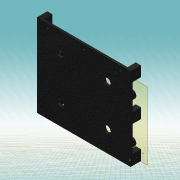
# Autodesk Inventor part: Down
Saved by Autodesk Inventor 2019 (Build 230136000, 136)
## iProperties
Created: 2024-12-30
Part Number: Down
Material: Nylon, molybdenum disulphide
Document SubType Name: Modeling
Designer: Familia CS
Density: 1.13 g/cm^3
Appearance: Black Cast
Author: Familia CS
Autodesk Inventor part; units mm, degrees
ref_plane "YZ Plane" through (0, 0, 0) normal (1, 0, 0) x (0, 1, 0)
ref_plane "XZ Plane" through (0, 0, 0) normal (0, 1, 0) x (-1, 0, 0)
ref_plane "XY Plane" through (0, 0, 0) normal (0, 0, 1) x (1, 0, 0)
ref_plane "Work Plane1" through (0, 0, 0) normal (0, 0, 1) x (1, 0, 0)
sketch "Sketch1" plane through (0, 0, 0) normal (0, 0, 1) x (1, 0, 0)
  circle A0 centre (-10, 5) radius 2 projected
  circle A1 centre (-80, 5) radius 2.426 projected
  circle A2 centre (-10, 45) radius 2 projected
  circle A3 centre (-80, 45) radius 2 projected
  circle A4 centre (-10, 5) radius 4
  circle A5 centre (-80, 5) radius 4
  circle A6 centre (-10, 45) radius 4
  circle A7 centre (-80, 45) radius 4
  point P0 (0, 0)
  dimension "d0" = 8
  dimension "d1" = 8
  dimension "d2" = 8
  dimension "d3" = 8
  constraints: 4 centre point, 4 coincident
  measures "d0" diameter of A4
  measures "d1" diameter of A5
  measures "d2" diameter of A6
  measures "d3" diameter of A7
extrude "Extrusion1" add sketch "Sketch1" along normal blind 10 contours A0 | A1 | A2 | A3 | A4 | A5 | A6 | A7
sketch "Sketch2" plane through (-10, 5, 10) normal (0, 0, 1) x (1, 0, 0)
  circle A0 centre (0, 0) radius 4 projected
  circle A1 centre (0, 0) radius 0.75
  circle A2 centre (-70, 0) radius 4 projected
  circle A3 centre (-70, 0) radius 0.75
  circle A4 centre (0, 40) radius 4 projected
  circle A5 centre (0, 40) radius 0.75
  circle A6 centre (-70, 40) radius 4 projected
  circle A7 centre (-70, 40) radius 0.75
  point P0 (10, -5)
  dimension "d6" = 1.5
  dimension "d7" = 1.5
  dimension "d8" = 1.5
  dimension "d9" = 1.5
  constraints: 4 centre point, 4 coincident
  measures "d6" diameter of A1
  measures "d7" diameter of A3
  measures "d8" diameter of A5
  measures "d9" diameter of A7
extrude "Extrusion2" cut sketch "Sketch2" against normal blind 10 contours A1 | A3 | A5 | A7
sketch "Sketch3" plane through (-10, 5, 10) normal (0, 0, 1) x (1, 0, 0)
  line L0 (-75, -10) -> (5, -10) projected
  line L1 (-80, 45) -> (-80, -5) projected
  line L2 (5, 50) -> (-75, 50) projected
  line L3 (10, -5) -> (10, 45) projected
  line L4 (-80.5, -10.5) -> (10.5, -10.5)
  line L5 (10.5, -10.5) -> (10.5, 70)
  line L6 (10.5, 70) -> (-80.5, 70)
  line L7 (-80.5, 70) -> (-80.5, -10.5)
  constraints: 8 end point, 2 parallel, 1 horizontal, 1 perpendicular
extrude "Extrusion3" add sketch "Sketch3" along normal blind 2
sketch "Sketch4" plane through (-10, 5, 12) normal (0, 0, 1) x (1, 0, 0)
  line L0 (-80.5, 70) -> (10.5, 70)
  circle A0 centre (-12.25, 9.625) radius 3.25
  circle A1 centre (-57.75, 9.625) radius 3.25
  circle A2 centre (-12.25, 49.875) radius 3.25
  circle A3 centre (-57.75, 50.6331) radius 3.25
  point P0 (10, -5)
  point P1 (10.5, -10.5)
  dimension "d18" = 6.5
  dimension "d19" = 6.5
  dimension "d20" = 6.5
  dimension "d21" = 6.5
  constraints: 4 centre point, 2 end point
  measures "d18" diameter of A0
  measures "d19" diameter of A1
  measures "d20" diameter of A2
  measures "d21" diameter of A3
extrude "Extrusion4" cut sketch "Sketch4" against normal blind 2
sketch "Sketch5" plane through (0.5, -5.5, 10) normal (1, 0, 0) x (0, 0, -1)
  point P0 (10, 5.5)
sketch "Sketch6" plane through (0.5, -5.5, 10) normal (1, 0, 0) x (0, 0, -1)
  point P0 (10, 5.5)
sketch "Sketch7" plane through (0.5, -5.5, 10) normal (1, 0, 0) x (0, 0, -1)
  line L0 (0, 0) -> (0, 80.5) projected
  line L1 (0, 0) -> (8, 0)
  line L2 (8, 0) -> (8, 10)
  line L3 (8, 10) -> (0, 10)
  line L4 (0, 10) -> (0, 0)
  circle A0 centre (4, 5) radius 0.75
  point P0 (10, 5.5)
  dimension "d24" = 8
  dimension "d25" = 10
  dimension "d26" = 1.5
  constraints: 8 end point, 2 parallel, 1 centre point, 1 horizontal, 1 perpendicular
  measures "d24" distance of L3.end L2.end
  measures "d25" distance of L2.end L1.end
  measures "d26" diameter of A0
extrude "Extrusion5" add sketch "Sketch7" against normal blind 5
sketch "Sketch8" plane through (-90.5, -5.5, 12) normal (0, -1, 0) x (1, 0, 0)
  line L0 (86, -10) -> (86, -2) projected
  line L1 (86, -10) -> (76, -10)
  line L2 (76, -10) -> (76, -2)
  line L3 (76, -2) -> (86, -2)
  line L4 (86, -2) -> (86, -10)
  circle A0 centre (81, -6) radius 0.75
  point P0 (90.5, -12)
  dimension "d29" = 10
  dimension "d30" = 8
  dimension "d31" = 1.5
  constraints: 8 end point, 2 parallel, 1 centre point, 1 horizontal, 1 perpendicular
  measures "d29" distance of L2.end L3.end
  measures "d30" distance of L1.end L2.end
  measures "d31" diameter of A0
extrude "Extrusion6" add sketch "Sketch8" against normal blind 5
fillet "Fillet1" radius 1 1 edges at (-14, 5, 10)
sketch "Sketch9" plane through (-90.5, -5.5, 12) normal (0, -1, 0) x (1, 0, 0)
  line L0 (0, -2) -> (76, -2) projected
  line L1 (0, -2) -> (10, -2)
  line L2 (10, -2) -> (10, -10)
  line L3 (10, -10) -> (0, -10)
  line L4 (0, -10) -> (0, -2)
  circle A0 centre (5, -6) radius 0.75
  point P0 (90.5, -12)
  dimension "d35" = 10
  dimension "d36" = 8
  dimension "d37" = 1.5
  constraints: 8 end point, 2 parallel, 1 centre point, 1 horizontal, 1 perpendicular
  measures "d35" distance of L2.end L3.end
  measures "d36" distance of L1.end L2.end
  measures "d37" diameter of A0
extrude "Extrusion7" add sketch "Sketch9" against normal blind 5
sketch "Sketch10" plane through (-90.5, -5.5, 12) normal (-1, 0, 0) x (0, 0, 1)
  line L0 (-2, 5) -> (-2, 0) projected
  line L1 (-2, 5) -> (-10, 5)
  line L2 (-10, 5) -> (-10, 15)
  line L3 (-10, 15) -> (-2, 15)
  line L4 (-2, 15) -> (-2, 5)
  circle A0 centre (-6, 10) radius 0.75
  point P0 (-12, 5.5)
  point P1 (-2, 10)
  point P2 (-10, 10)
  dimension "d40" = 8
  dimension "d41" = 10
  dimension "d42" = 1.5
  constraints: 8 end point, 2 parallel, 1 centre point, 1 horizontal, 1 perpendicular
  measures "d40" distance of L2.end L3.end
  measures "d41" distance of L1.end L2.end
  measures "d42" diameter of A0
extrude "Extrusion8" add sketch "Sketch10" against normal blind 5
fillet "Fillet2" radius 1 1 edges at (-84, 5, 10)
sketch "Sketch11" plane through (-90.5, -5.5, 12) normal (0, -1, 0) x (1, 0, 0)
  line L0 (10, -2) -> (76, -2) projected
  line L1 (76, -2) -> (10, -2)
  circle A0 centre (43, -6) radius 0.75
  line L2 (43, -2) -> (38, -2)
  line L3 (38, -2) -> (38, -10)
  line L4 (38, -10) -> (48, -10)
  line L5 (48, -10) -> (48, -2)
  point P0 (90.5, -12)
  dimension "d47" = 1.5
  dimension "d48" = 5
  dimension "d49" = 8
  dimension "d50" = 10
  constraints: 10 end point, 3 perpendicular, 2 point on line, 1 centre point, 1 collinear, 1 midpoint
  measures "d47" diameter of A0
  measures "d48" distance of L2.start L2.end
  measures "d49" distance of L2.end L3.end
  measures "d50" distance of L3.end L4.end
extrude "Extrusion9" add sketch "Sketch11" against normal blind 5
sketch "Sketch12" plane through (-90.5, -5.5, 12) normal (-1, 0, 0) x (0, 0, 1)
  point P0 (-12, 5.5)
fillet "Fillet3" radius 1 2 edges at (-84, 45, 10) (-14, 45, 10)
sketch "Sketch13" plane through (-90.5, -5.5, 12) normal (-1, 0, 0) x (0, 0, 1)
  line L0 (-10, 0) -> (0, 0) projected
  line L1 (0, 0) -> (0, 80.5)
  circle A0 centre (-6, 40.25) radius 0.75
  line L2 (-10, 40.25) -> (-10, 45.25)
  line L3 (-10, 45.25) -> (-2, 45.25)
  line L4 (-2, 45.25) -> (-2, 35.25)
  line L5 (-2, 80.5) -> (-2, 15) projected
  line L6 (-2, 35.25) -> (-10, 35.25)
  line L7 (-10, 35.25) -> (-10, 40.25)
  point P0 (-12, 5.5)
  dimension "d56" = 1.5
  dimension "d57" = 5
  dimension "d58" = 8
  dimension "d59" = 10
  dimension "d60" = 8
  constraints: 12 end point, 2 perpendicular, 2 point on line, 2 vertical, 1 centre point
  measures "d56" diameter of A0
  measures "d57" distance of L2.start L2.end
  measures "d58" distance of L2.end L3.end
  measures "d59" distance of L3.end L4.end
  measures "d60" distance of L4.end L6.end
extrude "Extrusion10" add sketch "Sketch13" against normal blind 5
sketch "Sketch14" plane through (0.5, -5.5, 12) normal (1, 0, 0) x (0, 0, -1)
  line L0 (10, 35.25) -> (10, 45.25) projected
  circle A0 centre (6, 40.25) radius 0.75 projected
  circle A1 centre (6, 40.25) radius 0.75
  line L1 (10, 40.25) -> (10, 35.25)
  line L2 (10, 35.25) -> (2, 35.25)
  line L3 (2, 10) -> (2, 80.5) projected
  line L4 (2, 35.25) -> (2, 45.25)
  line L5 (2, 45.25) -> (10, 45.25)
  line L6 (10, 45.25) -> (10, 40.25)
  point P0 (12, 5.5)
  dimension "d63" = 1.5
  dimension "d65" = 8
  dimension "d66" = 10
  dimension "d67" = 8
  constraints: 10 end point, 2 collinear, 2 midpoint, 1 centre point, 1 coincident, 1 perpendicular, 1 point on line
  measures "d63" diameter of A1
  measures "d65" distance of L0.start L2.end
  measures "d66" distance of L2.end L4.end
  measures "d67" distance of L4.end L0.end
extrude "Extrusion11" add sketch "Sketch14" against normal blind 5
sketch "Sketch15" plane through (0.5, -5.5, 12) normal (1, 0, 0) x (0, 0, -1)
  line L0 (2, 80.5) -> (0, 80.5) projected
  line L1 (2, 80.5) -> (10, 80.5)
  line L2 (10, 80.5) -> (10, 70.5)
  line L3 (10, 70.5) -> (2, 70.5)
  line L4 (2, 70.5) -> (2, 80.5)
  circle A0 centre (6, 75.5) radius 0.75
  point P0 (12, 5.5)
  dimension "d70" = 8
  dimension "d71" = 10
  dimension "d73" = 1.5
  constraints: 8 end point, 2 parallel, 1 centre point, 1 horizontal, 1 perpendicular
  measures "d70" distance of L2.end L3.end
  measures "d71" distance of L1.end L2.end
  measures "d73" diameter of A0
extrude "Extrusion12" add sketch "Sketch15" against normal blind 5
sketch "Sketch16" plane through (-90.5, -5.5, 12) normal (-1, 0, 0) x (0, 0, 1)
  line L0 (-2, 80.5) -> (0, 80.5) projected
  line L1 (-10, 70.5) -> (-2, 70.5) projected
  line L2 (-2, 80.5) -> (-10, 80.5)
  line L3 (-10, 80.5) -> (-10, 70.5)
  line L4 (-10, 70.5) -> (-2, 70.5)
  line L5 (-2, 70.5) -> (-2, 80.5)
  circle A0 centre (-6, 75.5) radius 0.75 projected
  circle A1 centre (-6, 75.5) radius 0.75
  point P0 (-12, 5.5)
  constraints: 8 end point, 2 parallel, 1 centre point, 1 coincident, 1 horizontal, 1 perpendicular
extrude "Extrusion13" add sketch "Sketch16" against normal blind 5
sketch "Sketch17" plane through (-10, 5, 10) normal (0, 0, -1) x (-1, 0, 0)
  circle A0 centre (35, 66) radius 1.25
  circle A1 centre (70.5, 66) radius 1.25
  circle A2 centre (-0.5, 66) radius 1.25
  point P0 (-10, -5)
  point P1 (75.5, 70)
  dimension "d79" = 2.5
  dimension "d83" = 2.5
  dimension "d85" = 2.5
  constraints: 3 centre point
  measures "d79" diameter of A0
  measures "d83" diameter of A1
  measures "d85" diameter of A2
extrude "Extrusion14" cut sketch "Sketch17" against normal blind 2
sketch "Sketch18" plane through (-10, 5, 12) normal (0, 0, 1) x (1, 0, 0)
  point P0 (10, -5)
body "Solid1"
